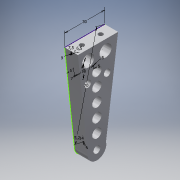
# Autodesk Inventor part: Radaufhängung
Saved by Autodesk Inventor 2018 (Build 220112000, 112)
## iProperties
Created: 2018-01-29
Part Number: Radaufhängung
Material: PC/ABS-Kunststoff
Document SubType Name: Modeling
Designer: Chris
Density: 0.357273 g/cm^3
Appearance: Schnee
Mass: 4.20281 g
Surface Area: 64.3362 cm^2
Volume: 11.7636 cm^3
Author: Chris
Autodesk Inventor part; units mm, degrees
ref_plane "YZ Plane" through (0, 0, 0) normal (1, 0, 0) x (0, 1, 0)
ref_plane "XZ Plane" through (0, 0, 0) normal (0, 1, 0) x (-1, 0, 0)
ref_plane "XY Plane" through (0, 0, 0) normal (0, 0, 1) x (1, 0, 0)
sketch "Skizze1" plane through (0, 0, 0) normal (1, 0, 0) x (0, 1, 0)
  line L0 (0, 0) -> (30, 0)
  line L1 (14.2054, 0) -> (14.2054, -68.1948) construction
  circle A0 centre (14.2054, -68.1948) radius 2.6
  circle A1 centre (14.2054, -68.1948) radius 7
  line L2 (30, 0) -> (20.9884, -66.4655)
  line L3 (0, 0) -> (7.2054, -68.1948)
  circle A2 centre (14.2054, -17.57) radius 3.5
  circle A3 centre (7.7054, -7.5) radius 4.5
  circle A4 centre (20.7054, -7.5) radius 4.5
  circle A5 centre (14.2054, -27.57) radius 3.5
  circle A6 centre (14.2054, -37.57) radius 3.5
  circle A7 centre (14.2054, -47.57) radius 3.5
  circle A8 centre (14.2054, -57.57) radius 3.5
  circle A9 centre (21.9208, -22.3731) radius 2.5
  circle A10 centre (7.3897, -22.3537) radius 2.5
  point P0 (11.3803, -37.5266)
  dimension "d0" = 30
  dimension "d32" = 70
  dimension "d34" = 5.2
  dimension "d35" = 14
  dimension "d36" = 7
  dimension "d42" = 9
  dimension "d43" = 7.5
  dimension "d44" = 6.5
  dimension "d47" = 10
  dimension "d54" = 5
  dimension "d58" = 5
  dimension "d59" = 5
  dimension "d60" = 5
  constraints: 11 centre point, 8 end point, 2 coincident, 2 point on circle, 2 point on line, 1 horizontal, 1 perpendicular, 1 symmetric about line, 1 vertical, 9 other
  measures "d0" distance of L0.start L0.end
  measures "d32" distance of L0.end L1.end
  measures "d34" diameter of A0
  measures "d35" diameter of A1
  measures "d36" diameter of A2
  measures "d42" diameter of A3
  measures "d43" distance from line of L0 A3.centre
  measures "d44" distance from line of L1 A3.centre
  measures "d47" distance of A2.centre A5.centre
  measures "d54" diameter of A9
  measures "d58" distance from line of L2 A9.centre
  measures "d59" diameter of A10
  measures "d60" distance from line of L3 A10.centre
extrude "Extrusion1" add sketch "Skizze1" along normal blind 10
sketch "Skizze3" plane through (0, 0, 0) normal (0, 0, 1) x (1, 0, 0)
  circle A0 centre (5, 8) radius 1.7
  line L0 (0, 0) -> (10, 0) projected
  circle A1 centre (5, 22) radius 1.7
  line L1 (0, 30) -> (10, 30) projected
  line L2 (10, 30) -> (10, 0) projected
  dimension "d24" = 3.4
  dimension "d25" = 8
  dimension "d26" = 3.4
  dimension "d27" = 8
  dimension "d28" = 5
  constraints: 2 centre point
  measures "d24" diameter of A0
  measures "d25" distance from line of L0 A0.centre
  measures "d26" diameter of A1
  measures "d27" distance from line of L1 A1.centre
  measures "d28" distance from line of L2 A0.centre
extrude "Extrusion2" cut sketch "Skizze3" against normal blind 11
